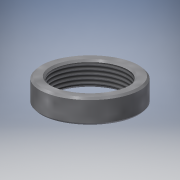
# Autodesk Inventor part: Component 38(Exhaust Pipe Ring)
Saved by Autodesk Inventor 2018 (Build 220112000, 112)
## iProperties
Created: 2023-04-01
Part Number: Component 38(Exhaust Pipe Ring)
Material: Generic
Document SubType Name: Modeling
Designer: Habib Mohamed
Density: 1 g/cm^3
Appearance: Flat - Polished Gray
Author: Habib Mohamed
Autodesk Inventor part; units mm, degrees
ref_plane "YZ Plane" through (0, 0, 0) normal (1, 0, 0) x (0, 1, 0)
ref_plane "XZ Plane" through (0, 0, 0) normal (0, 1, 0) x (-1, 0, 0)
ref_plane "XY Plane" through (0, 0, 0) normal (0, 0, 1) x (1, 0, 0)
sketch "Sketch1" plane through (0, 0, 0) normal (1, 0, 0) x (0, 1, 0)
  line L0 (0, 0) -> (3.594, 0) construction
  line L1 (3, 5.75) -> (3, 4.75)
  line L2 (3, 4.75) -> (2.75, 4.5)
  line L3 (2.75, 4.5) -> (0.25, 4.5)
  line L4 (0.25, 4.5) -> (0, 4.75)
  line L5 (0, 4.75) -> (0, 5.75)
  line L6 (2.75, 6) -> (3, 5.75)
  line L7 (2.75, 6) -> (0.25, 6)
  line L8 (0.25, 6) -> (0, 5.75)
  dimension "d3" = 3
  dimension "d4" = 4.5
  dimension "d6" = 6
  dimension "d7" = 0.25
  dimension "d8" = 0.25
  dimension "d9" = 0.25
  dimension "d10" = 0.25
  dimension "d11" = 0.25
  dimension "d12" = 0.25
  dimension "d13" = 0.25
  dimension "d14" = 0.25
  constraints: 18 end point, 2 horizontal, 1 parallel, 1 perpendicular, 1 point on line, 1 vertical
  measures "d3" distance between parallel lines of L5 L1
  measures "d4" distance between parallel lines of L0 L3
  measures "d6" distance between parallel lines of L0 L7
  measures "d7" horizontal distance of L1.start L6.start
  measures "d8" horizontal distance of L6.start L1.start
  measures "d9" horizontal distance of L5.end L7.end
  measures "d10" distance from line of L7 L5.end
  measures "d11" horizontal distance of L2.end L1.end
  measures "d12" horizontal distance of L1.end L2.end
  measures "d13" horizontal distance of L4.end L3.end
  measures "d14" horizontal distance of L4.end L3.end
revolve "Revolution1" add sketch "Sketch1" angle 360 about axis through (0, 0, 0) along (0, 1, 0)
thread "Thread1" size "M9x0.5" class "6H" standard "ANSI Metric M Profile" full length
body "Solid1"
